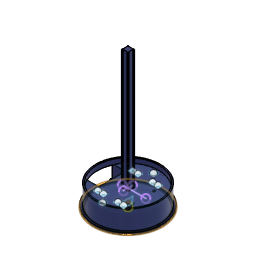
Paul's Lamp v24 (Autodesk Fusion 360 design; units mm, degrees)
Autodesk Fusion 360 part; units mm, degrees
sketch "Sketch1" plane through (0, 0, 0) normal (0, 1, 0) x (1, 0, 0) in component "Base"
  circle A0 centre (0, 0) radius 37.5
  circle A1 centre (0, 0) radius 35.25
  circle A2 centre (0, 0) radius 33.75
  dimension "d8" = 70.5
  dimension "d82" = -1.5
  constraint concentric A0 A1
  measures "d8" diameter of A1
  measures "d89" distance of A0.centre
  measures "d90" distance of A0.centre
sketch "Sketch1 (2)" plane through (0, 0, 0) normal (0, 1, 0) x (1, 0, 0) in component "Esp32 Module"
  line L0 (19.5768, -14.69) -> (-32.0432, -14.69)
  line L1 (-32.0432, -14.69) -> (-32.0432, 14.69)
  line L2 (-32.0432, 14.69) -> (19.5768, 14.69)
  line L3 (19.5768, 14.69) -> (19.5768, -14.69)
  line L4 (19.5768, -14.69) -> (-32.0432, 14.69) construction
  line L5 (-32.0432, -14.69) -> (19.5768, 14.69) construction
  circle A0 centre (0, 0) radius 35.25
  line L6 (-32.0432, 4.01) -> (-26.5332, 4.01)
  line L7 (-26.5332, 4.01) -> (-26.5332, -3.49)
  line L8 (-26.5332, -3.49) -> (-32.0432, -3.49)
  line L9 (-32.0432, -3.49) -> (-32.0432, 4.01)
  line L10 (-32.0432, 14.69) -> (-28.6432, 14.69) construction
  line L11 (-28.6432, 14.69) -> (-28.6432, 8.19) construction
  line L12 (-28.6432, 8.19) -> (-32.0432, 8.19) construction
  line L13 (-32.0432, 8.19) -> (-32.0432, 14.69) construction
  circle A1 centre (-28.6432, 8.19) radius 1.5
  line L14 (-32.0432, -8.19) -> (-28.6432, -8.19) construction
  line L15 (-28.6432, -8.19) -> (-28.6432, -14.69) construction
  line L16 (-28.6432, -14.69) -> (-32.0432, -14.69) construction
  line L17 (-32.0432, -14.69) -> (-32.0432, -8.19) construction
  circle A2 centre (-28.6432, -8.19) radius 1.5
  line L18 (-32.0432, -14.69) -> (-18.9432, -14.69) construction
  line L19 (-18.9432, -14.69) -> (-18.9432, -8.59) construction
  line L20 (-18.9432, -8.59) -> (-32.0432, -8.59) construction
  line L21 (-32.0432, -8.59) -> (-32.0432, -14.69) construction
  line L22 (-17.4432, -7.09) -> (-20.4432, -7.09)
  line L23 (-20.4432, -7.09) -> (-20.4432, -10.09)
  line L24 (-20.4432, -10.09) -> (-17.4432, -10.09)
  line L25 (-17.4432, -10.09) -> (-17.4432, -7.09)
  line L26 (-17.4432, -7.09) -> (-20.4432, -10.09) construction
  line L27 (-20.4432, -7.09) -> (-17.4432, -10.09) construction
  line L28 (19.5768, 14.69) -> (-17.4432, 14.69)
  line L29 (-17.4432, 14.69) -> (-17.4432, -14.69)
  line L30 (-17.4432, -14.69) -> (19.5768, -14.69)
  line L31 (19.5768, -14.69) -> (19.5768, 14.69)
  circle A3 centre (0, 0) radius 37.5
  line L32 (-32.0432, 14.69) -> (-34.503, 14.69)
  line L33 (-32.0432, -14.69) -> (-34.503, -14.69)
  arc A4 (-34.503, 14.69) -> (-34.503, -14.69) centre (-1.1733, 0) ccw
  line L34 (-17.4432, -13.5) -> (19.5768, -13.5)
  line L35 (19.5768, -13.5) -> (19.5768, -11.75)
  line L36 (19.5768, -11.75) -> (-17.4432, -11.75)
  line L37 (-17.4432, -11.75) -> (-17.4432, -13.5)
  line L38 (-6.2332, 0) -> (19.5768, 0) construction
  line L39 (-17.4432, 13.5) -> (19.5768, 13.5)
  line L40 (19.5768, 11.75) -> (-17.4432, 11.75)
  line L41 (-17.4432, 11.75) -> (-17.4432, 13.5)
  line L42 (19.5768, -14.69) -> (19.5768, 14.69)
  line L43 (-17.4432, 13.5) -> (-32.5624, 13.5)
  line L44 (-17.4432, 11.75) -> (-33.234, 11.75)
  line L45 (-17.4432, -11.75) -> (-33.234, -11.75)
  line L46 (-17.4432, -13.5) -> (-32.5624, -13.5)
  line L47 (19.5768, 0) -> (16.8768, 0)
  line L48 (16.8768, 0) -> (16.8768, -11.71)
  line L49 (16.8768, -11.71) -> (19.5768, -11.71)
  line L50 (19.5768, -11.71) -> (19.5768, 0)
  circle A5 centre (16.8768, -11.71) radius 1.25
  circle A6 centre (16.8768, 11.71) radius 1.25
  line L51 (19.5768, -13.5) -> (14.5768, -13.5)
  line L52 (14.5768, -13.5) -> (14.5768, 13.5)
  line L53 (14.5768, 13.5) -> (19.5768, 13.5)
  line L54 (19.5768, 13.5) -> (19.5768, -13.5)
  line L55 (14.5768, 13.5) -> (14.5867, 14.69)
  line L56 (14.5768, -13.5) -> (14.5349, -14.69)
  point P0 (-6.2332, 0)
  point P1 (-18.9432, -8.59)
  dimension "d9" = 51.62
  dimension "d10" = 29.38
  dimension "d15" = 5.51
  dimension "d16" = 7.5
  dimension "d17" = 18.18
  dimension "d18" = 3.4
  dimension "d19" = 6.5
  dimension "d20" = 3
  dimension "d21" = 3.4
  dimension "d22" = 6.5
  dimension "d23" = 3
  dimension "d24" = 13.1
  dimension "d25" = 6.1
  dimension "d26" = 3
  dimension "d27" = 3
  dimension "d32" = 1.75
  dimension "d33" = 1.19
  dimension "d99" = 2.7
  dimension "d100" = 11.71
  dimension "d101" = 2.5
  dimension "d104" = 5
  constraint horizontal L0
  constraint perpendicular L0 L1
  constraint parallel L0 L2
  constraint parallel L1 L3
  constraint coincident L4 P0
  constraint coincident L5 P0
  constraint coincident L1.end A0
  constraint coincident L0.end A0
  constraint horizontal L6
  constraint vertical L7
  constraint horizontal L8
  constraint vertical L9
  constraint coincident L1 L8.end
  constraint horizontal L10
  constraint vertical L11
  constraint horizontal L12
  constraint vertical L13
  constraint coincident L1.end L2.start
  constraint coincident L11.end L12.start
  constraint horizontal L14
  constraint vertical L15
  constraint horizontal L16
  constraint vertical L17
  constraint coincident L0.end L1.start
  constraint coincident L14.end L15.start
  constraint horizontal L18
  constraint vertical L19
  constraint horizontal L20
  constraint vertical L21
  constraint horizontal L22
  constraint perpendicular L22 L23
  constraint parallel L22 L24
  constraint parallel L23 L25
  constraint coincident L26 P1
  constraint coincident L27 P1
  constraint coincident P1 L19.end
  constraint horizontal L28
  constraint vertical L29
  constraint horizontal L30
  constraint vertical L31
  constraint coincident L0 L29.end
  constraint coincident L22.start L29
  constraint coincident A3 L32.end
  constraint perpendicular L1 L32
  constraint coincident A3 L33.end
  constraint perpendicular L21 L33
  constraint tangent A0 A4
  constraint horizontal L34
  constraint vertical L35
  constraint horizontal L36
  constraint vertical L37
  constraint coincident L31 L35.end
  constraint coincident L29 L36.end
  constraint coincident P0 L38.start
  constraint midpoint L3 L38.end
  constraint symmetric L0.start L38 L2.end
  constraint symmetric L2.end L38 L0.start
  constraint symmetric L34.start L38 L39.start
  constraint symmetric L34.end L38 L39.end
  constraint symmetric L35.end L38 L40.start
  constraint symmetric L36.end L38 L40.end
  constraint coincident A0 L43.end
  constraint perpendicular L41 L43
  constraint coincident A0 L44.end
  constraint perpendicular L13 L44
  constraint coincident A0 L45.end
  constraint perpendicular L21 L45
  constraint coincident A0 L46.end
  constraint perpendicular L17 L46
  constraint horizontal L47
  constraint vertical L48
  constraint horizontal L49
  constraint vertical L50
  constraint coincident L48.end L49.start
  constraint symmetric L38 A5 A6
  constraint horizontal L51
  constraint vertical L52
  constraint horizontal L53
  constraint vertical L54
  constraint coincident L2 L55.end
  constraint coincident L30 L56.end
  measures "d9" distance of L1.end L2.end
  measures "d10" distance of L0.end L1.end
  measures "d15" distance of L6.start L6.end
  measures "d16" distance of L6.start L8.end
  measures "d17" distance of L2 L8
  measures "d18" distance of L1.end L10.end
  measures "d19" distance of L1.end L12.end
  measures "d20" diameter of A1
  measures "d21" distance of L14.start L14.end
  measures "d22" distance of L14.start L0.end
  measures "d23" diameter of A2
  measures "d24" distance of L0.end L18.end
  measures "d25" distance of L0.end L20.end
  measures "d26" distance of L23.end L24.end
  measures "d27" distance of L22.end L23.end
  measures "d32" distance of L34.start L36.end
  measures "d33" distance of L0 L34
  measures "d99" distance of L38.end L47.end
  measures "d100" distance of L38.end L49.end
  measures "d101" diameter of A5
  measures "d104" distance of L34.end L51.end
extrude "Extrude1" add sketch "Sketch1 (2)" along normal blind 2 contours L0 L2 L3 A0 L28 L30 L31 L35 L42 L50 L54 | L0 L3 L30 L31 L34 L42 L51 L56 | L0 L29 L30 L34 L56 | L3 L31 L34 L35 L36 L42 A5 L51 L52 L54 | L29 L34 L36 L37 L52 | L3 L31 L36 L42 L49 A5 L54 | A0 A3 L32 L33 | L3 L31 L36 L40 L42 L47 L48 A5 A6 L52 L54 | L25 L29 L36 L40 L52 | L3 L31 L42 L47 L48 L49 L50 A5 L54 | L36 A5 | L36 L48 L49 A5 | L3 L31 L39 L40 L42 A6 L52 L53 L54 | L29 L39 L40 L41 L52 | L48 L49 A5 | L40 A6 | L40 A6 | L2 L3 L28 L31 L39 L42 L53 L55 | L2 L28 L29 L39 L55 picked at (-2.6137, 21.4253) picked at (16.2295, -14.2933) picked at (3.8895, -13.8967) picked at (19.048, -12.5093) picked at (3.9035, -12.9167) picked at (19.0934, -11.7278) picked at (-31.2352, 17.761) picked at (17.8889, 3.502) picked at (3.9035, -2.3633) picked at (17.8361, -3.4909) picked at (16.6279, -12.1266) picked at (16.8163, -10.8811) picked at (19.048, 12.5093) picked at (-6.7699, 12.3333) picked at (17.1673, -10.9312) picked at (16.6723, 12.0997) picked at (16.7519, 11.3392) picked at (16.2468, 13.8967) picked at (3.9068, 14.2933) makes body 1 in component "Esp32 Module"
extrude "Extrude2" add sketch "Sketch1 (2)" along normal blind 6.73 contours L0 L2 L3 A0 L28 L30 L31 L35 L42 L50 L54 picked at (-2.6137, 21.4253) bodies 1 in component "Esp32 Module"
ref_plane "WorkPlane1" through (1.6034, 6.73, 0) normal (0, 1, 0) x (1, 0, 0) in component "Esp32 Module"
extrude "Extrude3" add sketch "Sketch1 (2)" along normal blind 17.73 and the other way blind -6.73 separate body contours L0 L2 L3 A0 L28 L30 L31 L35 L42 L50 L54 | L0 L3 L30 L31 L34 L42 L51 L56 | L0 L29 L30 L34 L56 | L3 L31 L34 L35 L36 L42 A5 L51 L52 L54 | L0 L1 L29 L46 | L29 L34 L36 L37 L52 | L3 L31 L36 L42 L49 A5 L54 | L1 A0 L46 | L1 L29 L37 L45 L46 | L3 L31 L36 L40 L42 L47 L48 A5 A6 L52 L54 | L25 L29 L36 L40 L52 | L3 L31 L42 L47 L48 L49 L50 A5 L54 | L36 A5 | L36 L48 L49 A5 | L1 A0 L45 L46 | L1 L6 L7 L8 L22 L23 L24 L29 L44 L45 | L3 L31 L39 L40 L42 A6 L52 L53 L54 | L29 L39 L40 L41 L52 | L48 L49 A5 | L1 A0 L9 L44 L45 | L1 L2 L29 L43 | L1 A0 L43 | L22 L23 L24 L25 L29 | L40 A6 | L40 A6 | L1 L29 L41 L43 L44 | L2 L3 L28 L31 L39 L42 L53 L55 | L2 L28 L29 L39 L55 | L1 L6 L7 L8 L9 | L1 A0 L43 L44 | A1 | A2 picked at (-2.6137, 21.4253) picked at (16.2295, -14.2933) picked at (3.8895, -13.8967) picked at (19.048, -12.5093) picked at (-22.3099, -14.2933) picked at (3.9035, -12.9167) picked at (19.0934, -11.7278) picked at (-32.3333, -13.6329) picked at (-27.1765, -12.3333) picked at (17.8889, 3.502) picked at (3.9035, -2.3633) picked at (17.8361, -3.4909) picked at (16.6279, -12.1266) picked at (16.8163, -10.8811) picked at (-32.2943, -12.7236) picked at (-20.4732, 2.89) picked at (19.048, 12.5093) picked at (-6.7699, 12.3333) picked at (17.1673, -10.9312) picked at (-33.085, 0.9713) picked at (-27.1765, 13.8967) picked at (-32.3333, 13.6329) picked at (-18.4432, -9.09) picked at (16.6723, 12.0997) picked at (16.7519, 11.3392) picked at (-22.3099, 12.9167) picked at (16.2468, 13.8967) picked at (3.9068, 14.2933) picked at (-30.2065, 1.51) picked at (-32.2943, 12.7236) picked at (-28.8632, 9.154) picked at (-28.4979, -7.226) makes body 2 in component "Esp32 Module"
extrude "Extrude4" cut sketch "Sketch1 (2)" along normal blind 6.73 and the other way blind -15.73 contours L3 L31 L34 L35 L36 L42 A5 L51 L52 L54 | L29 L34 L36 L37 L52 | L36 A5 | L3 L31 L39 L40 L42 A6 L52 L53 L54 | L29 L39 L40 L41 L52 | L40 A6 picked at (19.048, -12.5093) picked at (3.9035, -12.9167) picked at (16.6279, -12.1266) picked at (19.048, 12.5093) picked at (-6.7699, 12.3333) picked at (16.6723, 12.0997) bodies 2 in component "Esp32 Module"
extrude "Extrude5" cut sketch "Sketch1 (2)" along normal blind 15.73 and the other way blind -6.73 contours L1 L29 L37 L45 L46 | L1 A0 L45 L46 | L1 L29 L41 L43 L44 | L1 A0 L43 L44 picked at (-27.1765, -12.3333) picked at (-32.2943, -12.7236) picked at (-22.3099, 12.9167) picked at (-32.2943, 12.7236) bodies 2 in component "Esp32 Module"
sketch "Sketch1 (3)" plane through (0, 0, 0) normal (0, 1, 0) x (1, 0, 0) in component "Tower"
  line L0 (-3, 3) -> (3, 3)
  line L1 (3, 3) -> (3, -3)
  line L2 (3, -3) -> (-3, -3)
  line L3 (-3, -3) -> (-3, 3)
  line L4 (-3, 3) -> (3, -3) construction
  line L5 (3, 3) -> (-3, -3) construction
  line L6 (-3.5, -3.5) -> (-2.5, -3.5)
  line L7 (-2.5, -3.5) -> (-2.5, -2.5)
  line L8 (-2.5, -2.5) -> (-3.5, -2.5)
  line L9 (-3.5, -2.5) -> (-3.5, -3.5)
  line L10 (-3.5, -3.5) -> (-2.5, -2.5) construction
  line L11 (-2.5, -3.5) -> (-3.5, -2.5) construction
  line L12 (0, 0) -> (0, -3) construction
  line L13 (0, 0) -> (3, 0) construction
  line L14 (2.5, -3.5) -> (2.5, -2.5)
  line L15 (2.5, -2.5) -> (3.5, -2.5)
  line L16 (3.5, -2.5) -> (3.5, -3.5)
  line L17 (3.5, -3.5) -> (2.5, -3.5)
  line L18 (3.5, 3.5) -> (2.5, 3.5)
  line L19 (2.5, 3.5) -> (2.5, 2.5)
  line L20 (2.5, 2.5) -> (3.5, 2.5)
  line L21 (3.5, 2.5) -> (3.5, 3.5)
  line L22 (-2.5, 3.5) -> (-2.5, 2.5)
  line L23 (-2.5, 2.5) -> (-3.5, 2.5)
  line L24 (-3.5, 2.5) -> (-3.5, 3.5)
  line L25 (-3.5, 3.5) -> (-2.5, 3.5)
  point P0 (-3, -3)
  dimension "d48" = 6
  dimension "d49" = 6
  dimension "d89" = 1
  dimension "d90" = 1
  constraint horizontal L0
  constraint perpendicular L0 L1
  constraint parallel L0 L2
  constraint parallel L1 L3
  constraint coincident L4 L12.start
  constraint coincident L5 L12.start
  constraint coincident L12.start L13.start
  constraint horizontal L6
  constraint perpendicular L6 L7
  constraint parallel L6 L8
  constraint parallel L7 L9
  constraint coincident L10 P0
  constraint coincident L11 P0
  constraint coincident P0 L2.end
  constraint midpoint L2 L12.end
  constraint midpoint L1 L13.end
  constraint symmetric L6.start L12 L16.end
  constraint symmetric L6.end L12 L14.start
  constraint symmetric L7.end L12 L14.end
  constraint symmetric L8.end L12 L15.end
  constraint symmetric L6.start L13 L24.end
  constraint symmetric L6.end L13 L22.start
  constraint symmetric L7.end L13 L22.end
  constraint symmetric L8.end L13 L23.end
  constraint symmetric L13 L14.start L18.end
  constraint symmetric L13 L14.end L19.end
  constraint symmetric L13 L15.end L20.end
  constraint symmetric L13 L16.end L18.start
  measures "d48" distance of L1.end P0
  measures "d49" distance of L0.end L1.end
  measures "d89" distance of L7.end L8.end
  measures "d90" distance of L6.end L7.end
extrude "Extrude1'" add sketch "Sketch1 (3)" along normal blind 150 and the other way blind -17.5 separate body contours L0 L3 L22 L23 | L0 L1 L2 L3 L7 L8 L14 L15 L19 L20 L22 L23 | L0 L1 L19 L20 | L2 L3 L7 L8 | L1 L2 L14 L15 picked at (-2.6667, 2.6667) picked at (-0.8333, -0.8333) picked at (2.8333, 2.6667) picked at (-2.6667, -2.8333) picked at (2.8333, -2.6667) makes body 3 in component "Tower"
sketch "Sketch1 (4)" plane through (0, 0, 0) normal (0, 1, 0) x (1, 0, 0) in component "Lens"
  circle A0 centre (0, 0) radius 37.5
  circle A1 centre (0, 0) radius 35.5
  dimension "d54" = 75
  constraint coincident A0.centre A1.centre
  measures "d54" diameter of A0
extrude "Extrude1''" add sketch "Sketch1 (4)" along normal blind 160 and the other way blind -158 separate body contours A1 picked at (5.3909, 6.76) makes body 4 in component "Lens"
extrude "Extrude2'" add sketch "Sketch1 (4)" along normal blind 160 and the other way blind -2 contours A0 picked at (36.6937, -1.863) bodies 4 in component "Lens"
extrude "Extrude6" cut sketch "Sketch1 (2)" along normal blind 18 and the other way blind -5 contours A0 A3 L32 L33 A4 | L1 L6 L7 L8 L22 L23 L24 L29 L44 L45 | L1 A0 L9 L44 L45 | L22 L23 L24 L25 L29 | L1 L6 L7 L8 L9 | A1 | A2 picked at (-35.9457, 0) picked at (-20.4732, 2.89) picked at (-33.085, 0.9713) picked at (-18.4432, -9.09) picked at (-30.2065, 1.51) picked at (-28.8632, 9.154) picked at (-28.4979, -7.226) bodies 2 in component "Esp32 Module"
sketch "Sketch2" plane through (0, 0, 0) normal (1, 0, 0) x (0, 0, -1)
  line L0 (-4.9895, 1.2122) -> (5, 1.2122)
  line L1 (5, 1.2122) -> (5, 7.5)
  line L2 (5, 7.5) -> (-4.9895, 7.5)
  line L3 (-4.9895, 7.5) -> (-4.9895, 1.2122)
  line L4 (-4.9895, 1.2122) -> (5, 7.5) construction
  line L5 (5, 1.2122) -> (-4.9895, 7.5) construction
  point P0 (0.0052, 4.3561)
  constraint horizontal L0
  constraint perpendicular L0 L1
  constraint parallel L0 L2
  constraint parallel L1 L3
  constraint coincident L4 P0
  constraint coincident L5 P0
extrude "Extrude7" [suppressed] in component "Esp32 Module"
extrude "Extrude3'" cut sketch "Sketch2" along normal blind -41 and the other way blind 31 contours L0 L1 L2 L3 picked at (1.6702, 3.3081) bodies 4 in component "Lens"
extrude "Extrude8" cut sketch "Sketch1 (2)" along normal blind 19 contours L0 L1 L29 L46 | L1 A0 L46 | A0 A3 L32 L33 A4 | L1 L29 L37 L45 L46 | L1 A0 L45 L46 | L1 L2 L29 L43 | L1 A0 L43 | L1 L29 L41 L43 L44 | L1 A0 L43 L44 picked at (-22.3099, -14.2933) picked at (-32.3333, -13.6329) picked at (-35.9457, 0) picked at (-27.1765, -12.3333) picked at (-32.2943, -12.7236) picked at (-27.1765, 13.8967) picked at (-32.3333, 13.6329) picked at (-22.3099, 12.9167) picked at (-32.2943, 12.7236) bodies 2 in component "Esp32 Module"
extrude "Extrude1'''" add sketch "Sketch1" along normal blind 23 and the other way blind -17.5 separate body contours A1 picked at (-5.9961, 34.1405) makes body 5
extrude "Extrude9" cut sketch "Sketch1 (2)" along normal blind 5 contours L3 L31 L36 L42 L49 A5 L54 | L3 L31 L36 L40 L42 L47 L48 A5 A6 L52 L54 | L25 L29 L36 L40 L52 | L3 L31 L42 L47 L48 L49 L50 A5 L54 | L36 L48 L49 A5 | L48 L49 A5 | L40 A6 picked at (19.0934, -11.7278) picked at (17.8889, 3.502) picked at (3.9035, -2.3633) picked at (17.8361, -3.4909) picked at (16.8163, -10.8811) picked at (17.1673, -10.9312) picked at (16.7519, 11.3392) bodies 1 in component "Esp32 Module"
combine "Combine1" operation add target body 5 tool bodies 2 1
extrude "Extrude2''" [suppressed]
extrude "Extrude2'''" add sketch "Sketch1 (3)" along normal blind 150 and the other way blind -17.5 contours L0 L3 L22 L23 L24 L25 | L0 L3 L22 L23 | L0 L1 L18 L19 L20 L21 | L0 L1 L19 L20 | L2 L3 L7 L8 | L2 L3 L6 L7 L8 L9 | L1 L2 L14 L15 L16 L17 | L1 L2 L14 L15 picked at (-3, 3.3333) picked at (-2.6667, 2.6667) picked at (3.3333, 3) picked at (2.8333, 2.6667) picked at (-2.6667, -2.8333) picked at (-3, -3.3333) picked at (3.3333, -3) picked at (2.8333, -2.6667) bodies 3 in component "Tower"
extrude "Extrude3''" cut sketch "Sketch1 (2)" along normal blind 18 contours L36 A5 | L36 L48 L49 A5 | L48 L49 A5 | L40 A6 | L40 A6 picked at (16.6279, -12.1266) picked at (16.8163, -10.8811) picked at (17.1673, -10.9312) picked at (16.6723, 12.0997) picked at (16.7519, 11.3392) bodies 5
extrude "Extrude4'" cut sketch "Sketch1 (2)" along normal blind 3 contours L3 L31 L34 L35 L36 L42 A5 L51 L52 L54 | L3 L31 L36 L40 L42 L47 L48 A5 A6 L52 L54 | L3 L31 L42 L47 L48 L49 L50 A5 L54 | L3 L31 L39 L40 L42 A6 L52 L53 L54 picked at (19.048, -12.5093) picked at (17.8889, 3.502) picked at (17.8361, -3.4909) picked at (19.048, 12.5093) bodies 5
extrude "Extrude5'" add sketch "Sketch1 (2)" along normal blind 17 and the other way blind -6.72 contours L3 L31 L34 L35 L36 L42 A5 L51 L52 L54 | L3 L31 L39 L40 L42 A6 L52 L53 L54 picked at (19.048, -12.5093) picked at (19.048, 12.5093) bodies 5
sketch "Sketch3" plane through (0, 17.73, 0) normal (0, 1, 0) x (-1, 0, 0)
  circle A0 centre (-16.8768, 11.71) radius 1.25
  circle A1 centre (-16.8768, -11.71) radius 1.25
  arc A2 (30.3853, 14.69) -> (30.3853, -14.69) centre (0, 0) ccw
  line L0 (30.3853, -14.69) -> (17.4432, -14.69)
  line L1 (17.4432, -14.69) -> (17.4432, 14.69)
  line L2 (17.4432, 14.69) -> (30.3853, 14.69)
  line L3 (-16, 21) -> (-6, 21)
  line L4 (-6, 21) -> (-6, 17)
  line L5 (-6, 17) -> (-16, 17)
  line L6 (-16, 17) -> (-16, 21)
  circle A3 centre (-14, 19) radius 1.5
  circle A4 centre (-8, 19) radius 1.5
  line L7 (0, -5) -> (0, 4.9895)
  line L8 (16, 17) -> (16, 21)
  line L9 (6, 21) -> (6, 17)
  line L10 (6, 17) -> (16, 17)
  circle A5 centre (14, 19) radius 1.5
  circle A6 centre (8, 19) radius 1.5
  line L11 (16, 21) -> (6, 21)
  line L12 (6.2332, 0) -> (-19.5768, 0)
  line L13 (-16, -21) -> (-6, -21)
  line L14 (-6, -17) -> (-16, -17)
  line L15 (-6, -21) -> (-6, -17)
  line L16 (-16, -17) -> (-16, -21)
  circle A7 centre (-8, -19) radius 1.5
  circle A8 centre (-14, -19) radius 1.5
  line L17 (16, -17) -> (16, -21)
  line L18 (16, -21) -> (6, -21)
  line L19 (6, -17) -> (16, -17)
  circle A9 centre (8, -19) radius 1.5
  circle A10 centre (14, -19) radius 1.5
  line L20 (6, -21) -> (6, -17)
  circle A11 centre (0, 28) radius 3
  circle A12 centre (0, -28) radius 3
  dimension "d111" = 10
  dimension "d112" = 4
  dimension "d113" = 3
  dimension "d114" = 3
  dimension "d123" = 6
  constraint horizontal L3
  constraint vertical L4
  constraint horizontal L5
  constraint vertical L6
  constraint symmetric L3.start L7 L8.end
  constraint symmetric L3.end L7 L9.start
  constraint symmetric L4.end L7 L9.end
  constraint symmetric L5.end L7 L8.start
  constraint symmetric A3 L7 A5
  constraint symmetric A4 L7 A6
  constraint symmetric L3.start L12 L13.start
  constraint symmetric L3.end L12 L13.end
  constraint symmetric L4.end L12 L14.start
  constraint symmetric L5.end L12 L14.end
  constraint symmetric A3 L12 A8
  constraint symmetric A4 L12 A7
  constraint symmetric L8.start L12 L17.start
  constraint symmetric L9.start L12 L18.end
  constraint symmetric L8.end L12 L17.end
  constraint symmetric L9.end L12 L19.start
  constraint symmetric A5 L12 A10
  constraint symmetric A6 L12 A9
  constraint symmetric L12 A11 A12
  measures "d111" distance of L3.start L3.end
  measures "d112" distance of L3.start L5.end
  measures "d113" diameter of A3
  measures "d114" diameter of A4
  measures "d123" diameter of A11
extrude "Extrude6'" cut sketch "Sketch3" along normal blind 20 and the other way blind 25 contours A3 | A4 | A5 | A6 | A7 | A8 | A9 | A10 picked at (-14.1113, 19.4875) picked at (-7.5329, 18.7102) picked at (13.8887, 19.4875) picked at (8.4944, 18.2453) picked at (-7.5329, -19.2898) picked at (-14.0374, -18.5237) picked at (8.3832, -18.438) picked at (13.9626, -18.5237) bodies 5
extrude "Extrude7'" cut sketch "Sketch3" along normal blind -13 and the other way blind 18 contours L3 L4 L5 L6 | L8 L9 L10 L11 | L13 L14 L15 L16 | L17 L18 L19 L20 picked at (-11.8887, 17.1792) picked at (11.8887, 17.1792) picked at (-11.8887, -20.8208) picked at (11.8887, -20.8208) bodies 5
extrude "Extrude8'" cut sketch "Sketch3" along normal blind 4 and the other way blind 20 contours A11 | A12 picked at (-0.5, 28.9957) picked at (-0.5, -27.0043) bodies 5
combine "Combine1'" operation add target body 3 tool bodies 5 in component "Tower"
extrude "Extrude3'''" cut 1 faces at (-6.7699, 9.73, -11.75) along direction (0, 0, 1) blind 2 on bodies 3 bodies 3 in component "Tower"
extrude "Extrude4''" cut 1 faces at (-6.7699, 9.73, 11.75) along direction (0, 0, -1) blind 2 on bodies 3 bodies 3 in component "Tower"
extrude "Extrude5''" cut 2 faces at (14.5768, 12.73, -11.6667) (14.5768, 12.73, 11.6667) along direction (1, 0, 0) blind 0.5 on bodies 3 bodies 3 in component "Tower"
extrude "Extrude6''" cut 2 faces at (5.7368, 6.73, -14.2933) (5.7368, 6.73, 14.2933) along direction (0, 1, 0) blind 9 on bodies 3 bodies 3 in component "Tower"
extrude "Extrude7''" cut sketch "Sketch1 (2)" along normal blind 3 contours L0 L3 L30 L31 L34 L42 L51 L56 | L2 L3 L28 L31 L39 L42 L53 L55 picked at (16.2295, -14.2933) picked at (16.2468, 13.8967) bodies 3 in component "Tower"
component "Base" placed x (1, 0, 0) y (0, 1, 0) z (0, 0, 1) at (0, 0, 0)
component "Esp32 Module" placed x (1, 0, 0) y (0, 1, 0) z (0, 0, 1) at (0, 0, 0)
component "Tower" placed x (1, 0, 0) y (0, 1, 0) z (0, 0, 1) at (0, 0, 0)
component "Lens" placed x (1, 0, 0) y (0, 1, 0) z (0, 0, 1) at (0, 0, 0)
hidden bodies 4
equation "Base_dia = 75 mm"
equation "tolerance_base_to_lens = 0.5 mm"
equation "lens_thickness = 2 mm"
equation "thickness_bottom_of_base = 2 mm"
equation "esp_thickness = 4.73 mm"
equation "d8 = Base_dia - 2 * lens_thickness - tolerance_base_to_lens"
equation "d9 = esp_length"
equation "d10 = esp_width + 1 mm"
equation "esp_length = 51.62 mm"
equation "esp_width = 28.38 mm"
equation "usb_y = 7.5 mm"
equation "usb_x = 5.51 mm"
equation "d15 = usb_x"
equation "d16 = usb_y"
equation "d28 = thickness_bottom_of_base"
equation "d30 = esp_thickness + thickness_bottom_of_base"
equation "esp_pin_depth = 9 mm"
equation "d36 = thickness_bottom_of_base + esp_thickness + esp_pin_depth + 2 mm"
equation "d38 = -( thickness_bottom_of_base + esp_thickness )"
equation "d40 = thickness_bottom_of_base + esp_thickness"
equation "d42 = -( thickness_bottom_of_base + esp_thickness + esp_pin_depth )"
equation "d44 = esp_thickness + thickness_bottom_of_base + esp_pin_depth"
equation "d46 = -( esp_thickness + thickness_bottom_of_base )"
equation "d54 = Base_dia"
equation "d55 = -lens_thickness"
equation "d62 = -thickness_bottom_of_base"
equation "d100 = ( 23.42 / 2 ) * 1 mm"
